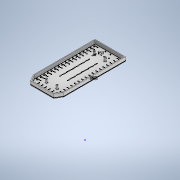
# Autodesk Inventor part: CaseBottomV2
Saved by Autodesk Inventor 2022 (Build 260153000, 153)
## iProperties
Created: 2021-05-25
Part Number: CaseBottomV2
Material: Generic
Document SubType Name: Modeling
Designer: Collin
Density: 1 g/cm^3
Appearance: Default
Author: Collin
Autodesk Inventor part; units mm, degrees
ref_plane "YZ Plane" through (0, 0, 0) normal (1, 0, 0) x (0, 1, 0)
ref_plane "XZ Plane" through (0, 0, 0) normal (0, 1, 0) x (-1, 0, 0)
ref_plane "XY Plane" through (0, 0, 0) normal (0, 0, 1) x (1, 0, 0)
sketch "Sketch1" plane through (0, 0, 0) normal (0, 1, 0) x (-1, 0, 0)
  line L0 (0, 0) -> (57.404, 0) construction
  line L1 (57.404, 0) -> (57.404, 120.904) construction
  line L2 (57.404, 120.904) -> (50.8, 132.334) construction
  line L3 (50.8, 132.334) -> (6.858, 132.334) construction
  line L4 (6.858, 132.334) -> (0, 121.158) construction
  line L5 (0, 121.158) -> (0, 0) construction
  circle A0 centre (4.318, 10.414) radius 0.51 construction
  circle A1 centre (4.318, 17.526) radius 0.51 construction
  circle A2 centre (4.318, 15.366) radius 0.55 construction
  circle A3 centre (4.318, 24.638) radius 0.51 construction
  circle A4 centre (4.318, 22.478) radius 0.55 construction
  circle A5 centre (6.858, 3.302) radius 0.51 construction
  circle A6 centre (6.858, 10.414) radius 0.51 construction
  circle A7 centre (6.858, 17.526) radius 0.51 construction
  circle A8 centre (4.318, 3.302) radius 0.51 construction
  circle A9 centre (4.318, 8.254) radius 0.55 construction
  circle A10 centre (18.542, 10.879) radius 1.27 construction
  circle A11 centre (9.398, 10.414) radius 0.51 construction
  circle A12 centre (9.398, 17.526) radius 0.51 construction
  circle A13 centre (18.034, 19.558) radius 2.15 construction
  circle A14 centre (9.398, 3.302) radius 0.51 construction
  circle A15 centre (23.622, 3.259) radius 1.995 construction
  circle A16 centre (21.082, 13.419) radius 0.8 construction
  circle A17 centre (26.162, 13.419) radius 0.8 construction
  circle A18 centre (53.086, 3.81) radius 0.51 construction
  circle A19 centre (48.006, 3.81) radius 0.51 construction
  circle A20 centre (50.546, 3.81) radius 0.51 construction
  circle A21 centre (53.086, 5.97) radius 0.55 construction
  circle A22 centre (50.546, 10.922) radius 0.51 construction
  circle A23 centre (53.086, 10.922) radius 0.51 construction
  circle A24 centre (48.006, 10.922) radius 0.51 construction
  circle A25 centre (48.006, 18.034) radius 0.51 construction
  circle A26 centre (50.546, 18.034) radius 0.51 construction
  circle A27 centre (53.086, 18.034) radius 0.51 construction
  circle A28 centre (53.086, 13.082) radius 0.55 construction
  circle A29 centre (31.242, 13.419) radius 0.8 construction
  circle A30 centre (36.322, 13.419) radius 0.8 construction
  circle A31 centre (33.782, 3.259) radius 1.995 construction
  circle A32 centre (39.37, 19.558) radius 2.15 construction
  circle A33 centre (38.862, 10.879) radius 1.27 construction
  circle A34 centre (53.086, 20.194) radius 0.55 construction
  circle A35 centre (21.082, 72.644) radius 0.5 construction
  circle A36 centre (21.082, 37.084) radius 0.5 construction
  circle A37 centre (36.322, 52.324) radius 0.5 construction
  circle A38 centre (48.006, 67.818) radius 0.51 construction
  circle A39 centre (55.626, 10.922) radius 0.51 construction
  circle A40 centre (55.626, 3.81) radius 0.51 construction
  circle A41 centre (55.626, 18.034) radius 0.51 construction
  circle A42 centre (1.778, 3.302) radius 0.51 construction
  circle A43 centre (1.778, 10.414) radius 0.51 construction
  circle A44 centre (1.778, 17.526) radius 0.51 construction
  circle A45 centre (1.778, 88.646) radius 0.51 construction
  circle A46 centre (4.318, 88.646) radius 0.51 construction
  circle A47 centre (9.398, 88.646) radius 0.51 construction
  circle A48 centre (6.858, 88.646) radius 0.51 construction
  circle A49 centre (21.082, 87.884) radius 0.5 construction
  circle A50 centre (55.626, 89.154) radius 0.51 construction
  circle A51 centre (53.086, 89.154) radius 0.51 construction
  circle A52 centre (50.546, 89.154) radius 0.51 construction
  circle A53 centre (48.006, 89.154) radius 0.51 construction
  circle A54 centre (36.322, 87.884) radius 0.5 construction
  circle A55 centre (53.086, 84.202) radius 0.55 construction
  circle A56 centre (36.322, 85.344) radius 0.5 construction
  circle A57 centre (4.318, 86.486) radius 0.55 construction
  circle A58 centre (21.082, 85.344) radius 0.5 construction
  circle A59 centre (9.398, 60.198) radius 0.51 construction
  circle A60 centre (21.082, 65.024) radius 0.5 construction
  circle A61 centre (21.082, 62.484) radius 0.5 construction
  circle A62 centre (21.082, 59.944) radius 0.5 construction
  circle A63 centre (9.398, 67.31) radius 0.51 construction
  circle A64 centre (21.082, 75.184) radius 0.5 construction
  circle A65 centre (21.082, 67.564) radius 0.5 construction
  circle A66 centre (21.082, 70.104) radius 0.5 construction
  circle A67 centre (9.398, 74.422) radius 0.51 construction
  circle A68 centre (21.082, 80.264) radius 0.5 construction
  circle A69 centre (21.082, 77.724) radius 0.5 construction
  circle A70 centre (21.082, 82.804) radius 0.5 construction
  circle A71 centre (9.398, 81.534) radius 0.51 construction
  circle A72 centre (50.546, 82.042) radius 0.51 construction
  circle A73 centre (48.006, 82.042) radius 0.51 construction
  circle A74 centre (36.322, 77.724) radius 0.5 construction
  circle A75 centre (36.322, 80.264) radius 0.5 construction
  circle A76 centre (36.322, 82.804) radius 0.5 construction
  circle A77 centre (50.546, 74.93) radius 0.51 construction
  circle A78 centre (48.006, 74.93) radius 0.51 construction
  circle A79 centre (36.322, 75.184) radius 0.5 construction
  circle A80 centre (36.322, 72.644) radius 0.5 construction
  circle A81 centre (36.322, 62.484) radius 0.5 construction
  circle A82 centre (36.322, 65.024) radius 0.5 construction
  circle A83 centre (36.322, 70.104) radius 0.5 construction
  circle A84 centre (36.322, 67.564) radius 0.5 construction
  circle A85 centre (50.546, 67.818) radius 0.51 construction
  circle A86 centre (50.546, 60.706) radius 0.51 construction
  circle A87 centre (48.006, 60.706) radius 0.51 construction
  circle A88 centre (36.322, 59.944) radius 0.5 construction
  circle A89 centre (4.318, 65.15) radius 0.55 construction
  circle A90 centre (4.318, 60.198) radius 0.51 construction
  circle A91 centre (4.318, 67.31) radius 0.51 construction
  circle A92 centre (6.858, 67.31) radius 0.51 construction
  circle A93 centre (6.858, 60.198) radius 0.51 construction
  circle A94 centre (6.858, 81.534) radius 0.51 construction
  circle A95 centre (6.858, 74.422) radius 0.51 construction
  circle A96 centre (4.318, 81.534) radius 0.51 construction
  circle A97 centre (4.318, 72.262) radius 0.55 construction
  circle A98 centre (4.318, 74.422) radius 0.51 construction
  circle A99 centre (4.318, 79.374) radius 0.55 construction
  circle A100 centre (53.086, 69.978) radius 0.55 construction
  circle A101 centre (53.086, 67.818) radius 0.51 construction
  circle A102 centre (53.086, 74.93) radius 0.51 construction
  circle A103 centre (53.086, 60.706) radius 0.51 construction
  circle A104 centre (53.086, 62.866) radius 0.55 construction
  circle A105 centre (53.086, 77.09) radius 0.55 construction
  circle A106 centre (53.086, 82.042) radius 0.51 construction
  circle A107 centre (1.778, 60.198) radius 0.51 construction
  circle A108 centre (1.778, 67.31) radius 0.51 construction
  circle A109 centre (1.778, 81.534) radius 0.51 construction
  circle A110 centre (1.778, 74.422) radius 0.51 construction
  circle A111 centre (55.626, 60.706) radius 0.51 construction
  circle A112 centre (55.626, 67.818) radius 0.51 construction
  circle A113 centre (55.626, 82.042) radius 0.51 construction
  circle A114 centre (55.626, 74.93) radius 0.51 construction
  circle A115 centre (36.322, 57.404) radius 0.5 construction
  circle A116 centre (21.082, 57.404) radius 0.5 construction
  circle A117 centre (4.318, 58.038) radius 0.55 construction
  circle A118 centre (1.778, 24.638) radius 0.51 construction
  circle A119 centre (1.778, 31.75) radius 0.51 construction
  circle A120 centre (4.318, 31.75) radius 0.51 construction
  circle A121 centre (4.318, 29.59) radius 0.55 construction
  circle A122 centre (6.858, 24.638) radius 0.51 construction
  circle A123 centre (6.858, 31.75) radius 0.51 construction
  circle A124 centre (6.858, 38.862) radius 0.51 construction
  circle A125 centre (4.318, 38.862) radius 0.51 construction
  circle A126 centre (1.778, 38.862) radius 0.51 construction
  circle A127 centre (4.318, 36.702) radius 0.55 construction
  circle A128 centre (9.398, 24.638) radius 0.51 construction
  circle A129 centre (21.082, 39.624) radius 0.5 construction
  circle A130 centre (21.082, 32.004) radius 0.5 construction
  circle A131 centre (21.082, 34.544) radius 0.5 construction
  circle A132 centre (9.398, 31.75) radius 0.51 construction
  circle A133 centre (9.398, 38.862) radius 0.51 construction
  circle A134 centre (1.778, 45.974) radius 0.51 construction
  circle A135 centre (6.858, 45.974) radius 0.51 construction
  circle A136 centre (4.318, 45.974) radius 0.51 construction
  circle A137 centre (4.318, 43.814) radius 0.55 construction
  circle A138 centre (9.398, 45.974) radius 0.51 construction
  circle A139 centre (21.082, 44.704) radius 0.5 construction
  circle A140 centre (21.082, 42.164) radius 0.5 construction
  circle A141 centre (21.082, 47.244) radius 0.5 construction
  circle A142 centre (55.626, 46.482) radius 0.51 construction
  circle A143 centre (53.086, 46.482) radius 0.51 construction
  circle A144 centre (50.546, 46.482) radius 0.51 construction
  circle A145 centre (55.626, 39.37) radius 0.51 construction
  circle A146 centre (53.086, 39.37) radius 0.51 construction
  circle A147 centre (50.546, 39.37) radius 0.51 construction
  circle A148 centre (53.086, 41.53) radius 0.55 construction
  circle A149 centre (48.006, 46.482) radius 0.51 construction
  circle A150 centre (48.006, 32.258) radius 0.51 construction
  circle A151 centre (50.546, 32.258) radius 0.51 construction
  circle A152 centre (55.626, 32.258) radius 0.51 construction
  circle A153 centre (53.086, 32.258) radius 0.51 construction
  circle A154 centre (48.006, 39.37) radius 0.51 construction
  circle A155 centre (53.086, 34.418) radius 0.55 construction
  circle A156 centre (53.086, 27.306) radius 0.55 construction
  circle A157 centre (36.322, 34.544) radius 0.5 construction
  circle A158 centre (36.322, 39.624) radius 0.5 construction
  circle A159 centre (36.322, 37.084) radius 0.5 construction
  circle A160 centre (36.322, 42.164) radius 0.5 construction
  circle A161 centre (36.322, 47.244) radius 0.5 construction
  circle A162 centre (36.322, 44.704) radius 0.5 construction
  circle A163 centre (36.322, 32.004) radius 0.5 construction
  circle A164 centre (55.626, 25.146) radius 0.51 construction
  circle A165 centre (53.086, 25.146) radius 0.51 construction
  circle A166 centre (48.006, 25.146) radius 0.51 construction
  circle A167 centre (50.546, 25.146) radius 0.51 construction
  circle A168 centre (36.322, 49.784) radius 0.5 construction
  circle A169 centre (21.082, 49.784) radius 0.5 construction
  circle A170 centre (53.086, 48.642) radius 0.55 construction
  circle A171 centre (4.318, 53.086) radius 0.51 construction
  circle A172 centre (4.318, 50.926) radius 0.55 construction
  circle A173 centre (6.858, 53.086) radius 0.51 construction
  circle A174 centre (9.398, 53.086) radius 0.51 construction
  circle A175 centre (21.082, 52.324) radius 0.5 construction
  circle A176 centre (55.626, 53.594) radius 0.51 construction
  circle A177 centre (53.086, 53.594) radius 0.51 construction
  circle A178 centre (48.006, 53.594) radius 0.51 construction
  circle A179 centre (50.546, 53.594) radius 0.51 construction
  circle A180 centre (1.778, 53.086) radius 0.51 construction
  circle A181 centre (53.086, 55.754) radius 0.55 construction
  circle A182 centre (36.322, 54.864) radius 0.5 construction
  circle A183 centre (21.082, 54.864) radius 0.5 construction
  circle A184 centre (55.626, 96.266) radius 0.51 construction
  circle A185 centre (53.086, 96.266) radius 0.51 construction
  circle A186 centre (53.086, 91.314) radius 0.55 construction
  circle A187 centre (50.546, 96.266) radius 0.51 construction
  circle A188 centre (48.006, 96.266) radius 0.51 construction
  circle A189 centre (36.322, 90.424) radius 0.5 construction
  circle A190 centre (6.858, 95.758) radius 0.51 construction
  circle A191 centre (9.398, 95.758) radius 0.51 construction
  circle A192 centre (21.082, 90.424) radius 0.5 construction
  circle A193 centre (4.318, 95.758) radius 0.51 construction
  circle A194 centre (4.318, 93.598) radius 0.55 construction
  circle A195 centre (1.778, 95.758) radius 0.51 construction
  circle A196 centre (55.626, 117.602) radius 0.51 construction
  circle A197 centre (53.086, 117.602) radius 0.51 construction
  circle A198 centre (48.006, 117.602) radius 0.51 construction
  circle A199 centre (50.546, 117.602) radius 0.51 construction
  circle A200 centre (53.086, 112.65) radius 0.55 construction
  circle A201 centre (53.086, 110.49) radius 0.51 construction
  circle A202 centre (48.006, 110.49) radius 0.51 construction
  circle A203 centre (50.546, 110.49) radius 0.51 construction
  circle A204 centre (55.626, 110.49) radius 0.51 construction
  circle A205 centre (39.37, 114.808) radius 2.15 construction
  circle A206 centre (9.398, 109.982) radius 0.51 construction
  circle A207 centre (9.398, 117.094) radius 0.51 construction
  circle A208 centre (18.034, 114.808) radius 2.15 construction
  circle A209 centre (9.398, 102.87) radius 0.51 construction
  circle A210 centre (53.086, 103.378) radius 0.51 construction
  circle A211 centre (48.006, 103.378) radius 0.51 construction
  circle A212 centre (50.546, 103.378) radius 0.51 construction
  circle A213 centre (53.086, 105.538) radius 0.55 construction
  circle A214 centre (55.626, 103.378) radius 0.51 construction
  circle A215 centre (4.318, 117.094) radius 0.51 construction
  circle A216 centre (4.318, 114.934) radius 0.55 construction
  circle A217 centre (6.858, 117.094) radius 0.51 construction
  circle A218 centre (4.318, 109.982) radius 0.51 construction
  circle A219 centre (6.858, 109.982) radius 0.51 construction
  circle A220 centre (6.858, 102.87) radius 0.51 construction
  circle A221 centre (4.318, 102.87) radius 0.51 construction
  circle A222 centre (4.318, 107.822) radius 0.55 construction
  circle A223 centre (4.318, 100.71) radius 0.55 construction
  circle A224 centre (1.778, 117.094) radius 0.51 construction
  circle A225 centre (1.778, 109.982) radius 0.51 construction
  circle A226 centre (1.778, 102.87) radius 0.51 construction
  circle A227 centre (53.086, 98.426) radius 0.55 construction
  circle A228 centre (10.16, 122.682) radius 0.51 construction
  circle A229 centre (17.272, 122.682) radius 0.51 construction
  circle A230 centre (24.384, 122.682) radius 0.51 construction
  circle A231 centre (38.608, 122.682) radius 0.51 construction
  circle A232 centre (31.496, 122.682) radius 0.51 construction
  circle A233 centre (53.086, 119.762) radius 0.55 construction
  circle A234 centre (45.72, 122.682) radius 0.51 construction
  circle A235 centre (24.384, 130.302) radius 0.51 construction
  circle A236 centre (17.272, 130.302) radius 0.51 construction
  circle A237 centre (22.224, 127.762) radius 0.55 construction
  circle A238 centre (17.272, 127.762) radius 0.51 construction
  circle A239 centre (31.496, 127.762) radius 0.51 construction
  circle A240 centre (29.336, 127.762) radius 0.55 construction
  circle A241 centre (24.384, 127.762) radius 0.51 construction
  circle A242 centre (31.496, 130.302) radius 0.51 construction
  circle A243 centre (17.272, 125.222) radius 0.51 construction
  circle A244 centre (24.384, 125.222) radius 0.51 construction
  circle A245 centre (31.496, 125.222) radius 0.51 construction
  circle A246 centre (38.608, 125.222) radius 0.51 construction
  circle A247 centre (36.448, 127.762) radius 0.55 construction
  circle A248 centre (38.608, 127.762) radius 0.51 construction
  circle A249 centre (38.608, 130.302) radius 0.51 construction
  circle A250 centre (45.72, 130.302) radius 0.51 construction
  circle A251 centre (45.72, 127.762) radius 0.51 construction
  circle A252 centre (43.56, 127.762) radius 0.55 construction
  circle A253 centre (45.72, 125.222) radius 0.51 construction
  circle A254 centre (10.16, 125.222) radius 0.51 construction
  circle A255 centre (10.16, 127.762) radius 0.51 construction
  circle A256 centre (10.16, 130.302) radius 0.51 construction
  circle A257 centre (15.112, 127.762) radius 0.55 construction
  circle A258 centre (8, 127.762) radius 0.55 construction
  circle A259 centre (4.318, 1.142) radius 0.55 construction
  line L6 (-0.0762, -0.0762) -> (57.4802, -0.0762)
  line L7 (57.4802, -0.0762) -> (57.4802, 120.9244)
  line L8 (57.4802, 120.9244) -> (50.844, 132.4102)
  line L9 (50.844, 132.4102) -> (6.8154, 132.4102)
  line L10 (6.8154, 132.4102) -> (-0.0762, 121.1795)
  line L11 (-0.0762, 121.1795) -> (-0.0762, -0.0762)
  line L12 (-1.6637, -1.6637) -> (59.0677, -1.6637)
  line L13 (59.0677, -1.6637) -> (59.0677, 121.3501)
  line L14 (59.0677, 121.3501) -> (51.7602, 133.9977)
  line L15 (51.7602, 133.9977) -> (5.9269, 133.9977)
  line L16 (5.9269, 133.9977) -> (-1.6637, 121.6278)
  line L17 (-1.6637, 121.6278) -> (-1.6637, -1.6637)
  circle A260 centre (39.37, 19.558) radius 1.905
  circle A261 centre (18.034, 19.558) radius 1.905
  circle A262 centre (18.034, 114.808) radius 1.905
  circle A263 centre (39.37, 114.808) radius 1.905
  point P0 (-98.298, 175.514)
  dimension "d0" = 0.0762
  dimension "d1" = 1.5875
  dimension "d6" = 3.81
  constraints: 264 centre point, 36 end point, 4 coincident, 3 equal radius, 2 horizontal, 2 vertical, 539 other
  measures "d0" distance between parallel lines of L5 L11
  measures "d1" distance between parallel lines of L11 L17
  measures "d6" diameter of A260
extrude "Extrusion1" add sketch "Sketch1" along normal blind 6.35 contours L17 L16 L15 L14 L13 L12
sketch "Sketch2" plane through (0, 0, 0) normal (0, -1, 0) x (1, 0, 0)
  line L0 (-59.0677, -1.6637) -> (-59.0677, 121.3501) projected
  line L1 (1.6637, -1.6637) -> (-59.0677, -1.6637) projected
  line L2 (1.6637, 121.6278) -> (1.6637, -1.6637) projected
  line L3 (-5.9269, 133.9977) -> (1.6637, 121.6278) projected
  line L4 (-51.7602, 133.9977) -> (-5.9269, 133.9977) projected
  line L5 (-59.0677, 121.3501) -> (-51.7602, 133.9977) projected
  line L6 (0.0762, -0.0762) -> (0.0762, 121.1795) projected
  line L7 (-57.4802, -0.0762) -> (0.0762, -0.0762) projected
  line L8 (-57.4802, 120.9244) -> (-57.4802, -0.0762) projected
  line L9 (-50.844, 132.4102) -> (-57.4802, 120.9244) projected
  line L10 (-6.8154, 132.4102) -> (-50.844, 132.4102) projected
  line L11 (0.0762, 121.1795) -> (-6.8154, 132.4102) projected
  point P0 (0, 0)
extrude "Extrusion2" add sketch "Sketch2" along normal blind 1.5875 contours L0 L5 L4 L3 L2 L1 | L7 L8 L9 L10 L11 L6
extrude "Extrusion3" add sketch "Sketch1" along normal up to surface (6.35 mm away) contours A260 | A261 | A262 | A263
sketch "Sketch3" plane through (-39.37, 6.35, 114.808) normal (0, 1, 0) x (1, 0, 0)
  circle A0 centre (0, 95.25) radius 1.905 projected
  circle A1 centre (0, 95.25) radius 1.27
  circle A2 centre (21.336, 95.25) radius 1.905 projected
  circle A3 centre (0, 0) radius 1.905 projected
  circle A4 centre (21.336, 0) radius 1.905 projected
  circle A5 centre (0, 0) radius 1.905 projected
  circle A6 centre (0, 0) radius 1.27
  circle A7 centre (21.336, 0) radius 1.905 projected
  circle A8 centre (21.336, 0) radius 1.27
  circle A9 centre (21.336, 95.25) radius 1.27
  point P0 (39.37, 114.808)
  dimension "d9" = 2.54
  constraints: 4 centre point, 4 coincident, 3 equal radius
  measures "d9" diameter of A1
extrude "Extrusion4" cut sketch "Sketch3" against normal up to surface (6.35 mm away) contours A1 | A6 | A8 | A9
equation "\"d10\" = d9"
body "Solid1"
